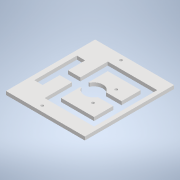
# Autodesk Inventor part: Etapa2Base
Saved by Autodesk Inventor 2021 (Build 250183000, 183)
## iProperties
Created: 2022-11-05
Part Number: Etapa2Base
Material: Genérico
Document SubType Name: Modeling
Designer: ivanm
Density: 1 g/cm^3
Appearance: Valor por defecto
Author: ivanm
Autodesk Inventor part; units mm, degrees
ref_plane "YZ Plane" through (0, 0, 0) normal (1, 0, 0) x (0, 1, 0)
ref_plane "XZ Plane" through (0, 0, 0) normal (0, 1, 0) x (-1, 0, 0)
ref_plane "XY Plane" through (0, 0, 0) normal (0, 0, 1) x (1, 0, 0)
sketch "Boceto1" plane through (0, 0, 0) normal (0, 1, 0) x (-1, 0, 0)
  line L0 (-352.8177, -763.3588) -> (-352.8177, -1023.3588) projected
  line L1 (-352.8177, -1023.3588) -> (-122.8177, -1023.3588) projected
  line L2 (-122.8177, -1023.3588) -> (-122.8177, -763.3588) projected
  line L3 (-122.8177, -763.3588) -> (-352.8177, -763.3588) projected
  circle A0 centre (-329.0452, -813.9623) radius 4 projected
  circle A1 centre (-329.0452, -973.9623) radius 4 projected
  circle A2 centre (-279.5292, -859.9623) radius 4 projected
  circle A3 centre (-212.5014, -779.1398) radius 4 projected
  circle A4 centre (-149.0452, -842.9623) radius 4 projected
  circle A5 centre (-149.0452, -944.9623) radius 4 projected
  circle A6 centre (-212.5014, -1008.7847) radius 4 projected
  circle A7 centre (-279.5292, -927.9623) radius 4 projected
  line L4 (-122.8177, -763.3588) -> (-352.8177, -763.3588)
  line L5 (-352.8177, -763.3588) -> (-352.8177, -1023.3588)
  line L6 (-352.8177, -1023.3588) -> (-122.8177, -1023.3588)
  line L7 (-122.8177, -1023.3588) -> (-122.8177, -763.3588)
  circle A8 centre (-329.0452, -973.9623) radius 4 projected
  circle A9 centre (-329.0452, -813.9623) radius 4 projected
  line L8 (-159.0452, -953.9623) -> (-139.0452, -953.9623) projected
  line L9 (-139.0452, -953.9623) -> (-139.0452, -833.9623) projected
  line L10 (-139.0452, -833.9623) -> (-159.0452, -833.9623) projected
  line L11 (-159.0452, -833.9623) -> (-159.0452, -883.9623) projected
  line L12 (-159.0452, -883.9623) -> (-199.0452, -883.9623) projected
  line L13 (-199.0452, -883.9623) -> (-199.0452, -803.9623) projected
  line L14 (-199.0452, -803.9623) -> (-339.0452, -803.9623) projected
  line L15 (-339.0452, -803.9623) -> (-339.0452, -983.9623) projected
  line L16 (-339.0452, -983.9623) -> (-199.0452, -983.9623) projected
  line L17 (-199.0452, -983.9623) -> (-199.0452, -903.9623) projected
  line L18 (-199.0452, -903.9623) -> (-159.0452, -903.9623) projected
  line L19 (-159.0452, -903.9623) -> (-159.0452, -953.9623) projected
  circle A10 centre (-149.0452, -944.9623) radius 4 projected
  circle A11 centre (-149.0452, -842.9623) radius 4 projected
  line L20 (-219.0452, -903.9623) -> (-219.0452, -963.9623) projected
  line L21 (-219.0452, -963.9623) -> (-319.0452, -963.9623) projected
  line L22 (-319.0452, -963.9623) -> (-319.0452, -903.9623) projected
  line L23 (-319.0452, -903.9623) -> (-270.958, -903.9623) projected
  arc A12 (-270.958, -903.9623) -> (-225.1323, -903.9623) centre (-248.0452, -893.9623) ccw projected
  line L24 (-225.1323, -903.9623) -> (-219.0452, -903.9623) projected
  line L25 (-219.0452, -883.9623) -> (-225.1323, -883.9623) projected
  arc A13 (-225.1323, -883.9623) -> (-270.958, -883.9623) centre (-248.0452, -893.9623) ccw projected
  line L26 (-270.958, -883.9623) -> (-319.0452, -883.9623) projected
  line L27 (-319.0452, -883.9623) -> (-319.0452, -823.9623) projected
  line L28 (-319.0452, -823.9623) -> (-219.0452, -823.9623) projected
  line L29 (-219.0452, -823.9623) -> (-219.0452, -883.9623) projected
  line L30 (-197.0452, -801.9623) -> (-197.0452, -881.9623)
  line L31 (-197.0452, -881.9623) -> (-161.0452, -881.9623)
  line L32 (-161.0452, -881.9623) -> (-161.0452, -831.9623)
  line L33 (-161.0452, -831.9623) -> (-137.0452, -831.9623)
  line L34 (-137.0452, -831.9623) -> (-137.0452, -955.9623)
  line L35 (-137.0452, -955.9623) -> (-161.0452, -955.9623)
  line L36 (-161.0452, -955.9623) -> (-161.0452, -905.9623)
  line L37 (-161.0452, -905.9623) -> (-197.0452, -905.9623)
  line L38 (-197.0452, -905.9623) -> (-197.0452, -985.9623)
  line L39 (-197.0452, -985.9623) -> (-341.0452, -985.9623)
  line L40 (-341.0452, -985.9623) -> (-341.0452, -801.9623)
  line L41 (-341.0452, -801.9623) -> (-197.0452, -801.9623)
  arc A14 (-272.2319, -905.9623) -> (-223.8584, -905.9623) centre (-248.0452, -893.9623) ccw
  line L42 (-272.2319, -905.9623) -> (-317.0452, -905.9623)
  line L43 (-317.0452, -905.9623) -> (-317.0452, -961.9623)
  line L44 (-317.0452, -961.9623) -> (-221.0452, -961.9623)
  line L45 (-221.0452, -961.9623) -> (-221.0452, -905.9623)
  line L46 (-221.0452, -905.9623) -> (-223.8584, -905.9623)
  arc A15 (-223.8584, -881.9623) -> (-272.2319, -881.9623) centre (-248.0452, -893.9623) ccw
  line L47 (-223.8584, -881.9623) -> (-221.0452, -881.9623)
  line L48 (-221.0452, -881.9623) -> (-221.0452, -825.9623)
  line L49 (-221.0452, -825.9623) -> (-317.0452, -825.9623)
  line L50 (-317.0452, -825.9623) -> (-317.0452, -881.9623)
  line L51 (-317.0452, -881.9623) -> (-272.2319, -881.9623)
  point P0 (0, 0)
  dimension "d0" = 2
  dimension "d1" = 2
  dimension "d2" = 2
  constraints: 52 end point, 4 point on circle, 2 centre point, 2 parallel, 1 horizontal, 1 perpendicular, 21 other
  measures "d0" distance between parallel lines of L13 L30
  measures "d1" radial gap between concentric circles of A12 A14
  measures "d2" radial gap between concentric circles of A13 A15
extrude "Extrusión1" add sketch "Boceto1" along normal blind 10 contours L3 L2 L1 L0 | A14 L46 L45 L44 L43 L42 | A15 L51 L50 L49 L48 L47
